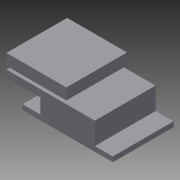
# Autodesk Inventor part: TeensyBLENunchukBundle
Saved by Autodesk Inventor 2015 SP1 (Build 190203100, 203)
## iProperties
Created: 2016-04-06
Part Number: TeensyBLENunchukBundle
Material: Generic
Document SubType Name: Modeling
Designer: doctor
Density: 1 g/cm^3
Appearance: Default
Author: doctor
Autodesk Inventor part; units mm, degrees
ref_plane "YZ Plane" through (0, 0, 0) normal (1, 0, 0) x (0, 1, 0)
ref_plane "XZ Plane" through (0, 0, 0) normal (0, 1, 0) x (-1, 0, 0)
ref_plane "XY Plane" through (0, 0, 0) normal (0, 0, 1) x (1, 0, 0)
sketch "Sketch1" plane through (0, 0, 0) normal (0, 0, 1) x (1, 0, 0)
  line L0 (0, 0) -> (36.3, 0)
  line L1 (36.3, 0) -> (36.3, -18)
  line L2 (36.3, -18) -> (0, -18)
  line L3 (0, -18) -> (0, 0)
  line L4 (-22.7, 2.1663) -> (17.3, 2.1663)
  line L5 (17.3, 2.1663) -> (17.3, 9.6663)
  line L6 (17.3, 9.6663) -> (-22.7, 9.6663)
  line L7 (-22.7, 9.6663) -> (-22.7, 2.1663)
  line L8 (-22.7, -4.6543) -> (0, -4.6543)
  line L9 (0, -4.6543) -> (0, 0)
  line L10 (0, 0) -> (-22.7, 0)
  line L11 (-22.7, 0) -> (-22.7, -4.6543)
  line L12 (36.3, -18) -> (48.3, -18)
  line L13 (48.3, -18) -> (48.3, -14.6921)
  line L14 (48.3, -14.6921) -> (36.3, -14.6921)
  line L15 (36.3, -14.6921) -> (36.3, -18)
  line L16 (0, -18) -> (-12, -18)
  line L17 (-12, -18) -> (-12, -14.6921)
  line L18 (-12, -14.6921) -> (0, -14.6921)
  line L19 (0, -14.6921) -> (0, -18)
  dimension "d0" = 36.3
  dimension "d1" = 18
  dimension "d2" = 40
  dimension "d3" = 7.5
  dimension "d4" = 59
  dimension "d5" = 71
  constraints: 40 end point, 10 parallel, 5 horizontal, 5 perpendicular, 1 coincident, 1 collinear
  measures "d0" distance of L1.end L2.end
  measures "d1" distance of L0.end L1.end
  measures "d2" distance of L6.end L5.end
  measures "d3" distance of L5.end L4.end
  measures "d4" distance between parallel lines of L1 L11
  measures "d5" distance between parallel lines of L11 L13
extrude "Extrusion1" add sketch "Sketch1" along normal blind 40.5
body "Solid1"
